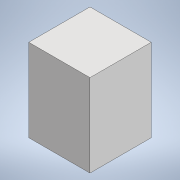
# Autodesk Inventor part: Joint_Bearings
Saved by Autodesk Inventor 2022.3 (Build 263350000, 350)
## iProperties
Created: 2023-03-29
Part Number: Joint_Bearings
Material: Generic
Document SubType Name: Modeling
Designer: Manuel Hueso Béjar
Density: 1 g/cm^3
Appearance: Default
Author: Manuel Hueso Béjar
Autodesk Inventor part; units mm, degrees
ref_plane "YZ Plane" through (0, 0, 0) normal (1, 0, 0) x (0, 1, 0)
ref_plane "XZ Plane" through (0, 0, 0) normal (0, 1, 0) x (-1, 0, 0)
ref_plane "XY Plane" through (0, 0, 0) normal (0, 0, 1) x (1, 0, 0)
sketch "Sketch1" plane through (0, 0, 0) normal (0, 1, 0) x (-1, 0, 0)
  line L0 (-25, -30) -> (25, -30)
  line L1 (25, -30) -> (25, 30)
  line L2 (25, 30) -> (-25, 30)
  line L3 (-25, 30) -> (-25, -30)
  line L4 (-25, -30) -> (25, 30) construction
  line L5 (25, -30) -> (-25, 30) construction
  point P0 (0, 0)
  dimension "d0" = 50
  dimension "d1" = 60
  constraints: 12 end point, 2 midpoint, 2 parallel, 1 horizontal, 1 perpendicular
  measures "d0" distance of L2.end L1.end
  measures "d1" distance of L1.end L0.end
extrude "Extrusion1" add sketch "Sketch1" along normal blind 53
sketch "Sketch2" plane through (-25, 0, 30) normal (0, 0, 1) x (1, 0, 0)
  line L0 (0, 0) -> (0, 53) projected
  line L1 (50, 0) -> (50, 53) projected
  line L2 (0, 53) -> (50, 53)
  line L3 (50, 53) -> (50, 49)
  line L4 (50, 49) -> (0, 49)
  line L5 (0, 49) -> (0, 53)
  line L6 (12.5, 49) -> (37.5, 49)
  line L7 (37.5, 49) -> (37.5, 57)
  line L8 (37.5, 57) -> (12.5, 57)
  line L9 (12.5, 57) -> (12.5, 49)
  line L10 (0, 53) -> (50, 53) projected
  line L11 (12.5, 49) -> (37.5, 57) construction
  line L12 (37.5, 49) -> (12.5, 57) construction
  line L13 (25, 49) -> (25, 11.5)
  line L14 (46, 11.5) -> (4, 11.5)
  line L15 (4, 11.5) -> (4, 49)
  line L16 (4, 49) -> (46, 49)
  line L17 (46, 49) -> (46, 11.5)
  line L18 (46, 11.5) -> (4, 49) construction
  line L19 (4, 11.5) -> (46, 49) construction
  point P0 (25, 0)
  point P1 (25, 53)
  point P2 (25, 30.25)
  point P3 (37.5, 49)
  point P4 (37.5, 53)
  point P5 (12.5, 53)
  point P6 (12.5, 49)
  dimension "d4" = 4
  dimension "d5" = 25
  dimension "d6" = 8
  dimension "d7" = 37.5
  dimension "d8" = 42
  constraints: 34 end point, 7 midpoint, 6 parallel, 3 horizontal, 3 perpendicular, 2 point on line, 1 vertical
  measures "d4" distance of L2.end L3.end
  measures "d5" distance of L8.end L7.end
  measures "d6" distance of L7.end L6.end
  measures "d7" distance of L13.start L13.end
  measures "d8" distance of L15.end L16.end
extrude "Extrusion2" cut sketch "Sketch2" against normal blind 51 contours L4 L13 L14 L15 | L2 L7 L4 L9 | L4 L17 L14 L13
sketch "Sketch3" plane through (25, 0, 30) normal (1, 0, 0) x (0, 0, -1)
  line L0 (30, 0) -> (12.5, 0)
  line L1 (12.5, 0) -> (47.5, 0)
  line L2 (0, 0) -> (60, 0) projected
  circle A0 centre (12.5, 0) radius 7.5
  circle A1 centre (47.5, 0) radius 7.5
  point P0 (55, 0)
  point P1 (40, 0)
  point P2 (20, 0)
  point P3 (5, 0)
  dimension "d11" = 17.5
  dimension "d12" = 35
  dimension "d13" = 15
  dimension "d14" = 15
  constraints: 4 end point, 2 centre point, 2 coincident, 1 horizontal, 1 point on line
  measures "d11" distance of L0.start L0.end
  measures "d12" distance of L0.end L1.end
  measures "d13" diameter of A0
  measures "d14" diameter of A1
extrude "Extrusion3" cut sketch "Sketch3" against normal blind 37 contours L0 L2 A0 | A1 L2 L1 picked at (17.141, 1.7601) picked at (45.1933, 4.395)
extrude "Extrusion4" add sketch "Sketch3" against normal blind 13 contours L0 L2 A0 | A1 L2 L1 picked at (17.141, 1.7601) picked at (45.1933, 4.395)
fillet "Fillet1" radius 4 11 edges at (25, 53, 0) (-25, 53, 0) (25, 26.5, 30) (-25, 26.5, 30) (25, 0, 0) (25, 26.5, -30) (0, 53, -30) (-25, 26.5, -30) (-25, 0, 0) (0, 0, 30) (0, 0, -30)
sketch "Sketch4" plane through (-25, 4, 26) normal (-1, 0, 0) x (0, 0, 1)
  line L0 (-35, -15) -> (-17, -15)
  line L1 (-17, -15) -> (-17, 7)
  line L2 (-17, 7) -> (-35, 7)
  line L3 (-35, 7) -> (-35, -15)
  line L4 (-35, -15) -> (-17, 7) construction
  line L5 (-17, -15) -> (-35, 7) construction
  point P0 (-26, -4)
  dimension "d20" = 18
  dimension "d21" = 22
  constraints: 12 end point, 2 midpoint, 2 parallel, 1 horizontal, 1 perpendicular
  measures "d20" distance of L2.end L1.end
  measures "d21" distance of L1.end L0.end
extrude "Extrusion5" cut sketch "Sketch4" against normal through all
sketch "Sketch5" plane through (0, 53, 0) normal (0, 1, 0) x (1, 0, 0)
  line L0 (-12.5, 21) -> (12.5, 21) projected
  line L1 (0, 21) -> (0, -21)
  line L2 (0, 21) -> (42, 21) construction
  line L3 (15.5, 15.5) -> (-15.5, 15.5)
  line L4 (-15.5, 15.5) -> (-15.5, -15.5)
  line L5 (-15.5, -15.5) -> (15.5, -15.5)
  line L6 (15.5, -15.5) -> (15.5, 15.5)
  line L7 (15.5, 15.5) -> (-15.5, -15.5) construction
  line L8 (-15.5, 15.5) -> (15.5, -15.5) construction
  point P0 (0, 0)
  dimension "d24" = 42
  dimension "d25" = 90
  dimension "d26" = 31
  dimension "d27" = 31
  constraints: 16 end point, 3 midpoint, 2 horizontal, 2 parallel, 2 perpendicular, 1 vertical
  measures "d24" distance of L1.start L1.end
  measures "d25" angle of L1 L2
  measures "d26" distance of L5.end L4.end
  measures "d27" distance of L4.end L3.end
hole "Hole1" at (15.5, 53, 15.5) at (15.5, 53, -15.5) at (-15.5, 53, -15.5) at (-15.5, 53, 15.5) direction (0, -1, 0) diameter 2.4 depth 4 countersink diameter 4 countersink angle 90
body "Solid1"
